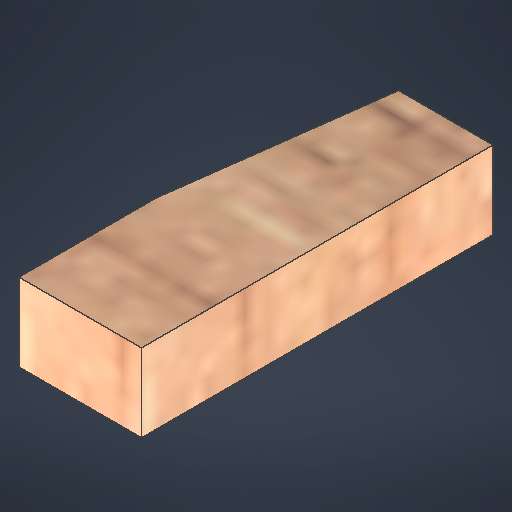
# Autodesk Inventor part: Stop Skiba
Saved by Autodesk Inventor 2027.1 (Build 311270010, 270A)
## iProperties
Created: 2025-11-09
Part Number: Stop Skiba
Material: Generic
Document SubType Name: Modeling
Designer: Nick
Density: 1 g/cm^3
Appearance: Birch - Natural Polished
Mass: 1.69348 g
Surface Area: 10.1101 cm^2
Volume: 1.69348 cm^3
Author: Nick
Autodesk Inventor part; units mm, degrees
ref_plane "YZ Plane" through (0, 0, 0) normal (1, 0, 0) x (0, 1, 0)
ref_plane "XZ Plane" through (0, 0, 0) normal (0, 1, 0) x (-1, 0, 0)
ref_plane "XY Plane" through (0, 0, 0) normal (0, 0, 1) x (1, 0, 0)
sketch "Sketch4" plane through (0, 0, 0) normal (0, 1, 0) x (-1, 0, 0)
  line L0 (5.0499, 10.8071) -> (-4.9501, 10.8071)
  line L1 (-4.9501, 10.8071) -> (-4.9501, -14.1929)
  line L2 (-4.9501, -14.1929) -> (5.0499, -14.1929)
  line L3 (5.0499, -14.1929) -> (5.0499, 10.8071)
  line L4 (5.0499, 3.3071) -> (-4.9501, 3.3071)
  line L5 (-4.9501, 3.3071) -> (-4.9501, 14.4921)
  line L6 (-4.9501, 14.4921) -> (5.0499, 14.4921)
  line L7 (5.0499, 14.4921) -> (5.0499, 3.3071)
  line L8 (5.0499, 3.3071) -> (2.7459, -14.1929)
  point P0 (0, 0)
  dimension "d12" = 10
  dimension "d13" = 25
  dimension "d14" = 10
  constraints: 18 end point, 4 parallel, 2 horizontal, 2 perpendicular, 1 point on line
  measures "d12" distance of L2.end L1.end
  measures "d13" distance of L1.end L0.end
  measures "d14" distance of L6.start L7.start
extrude "Extrusion7" add sketch "Sketch4" along normal blind 6.35 contours L3 L4 L1 L0 | L0 L5 L6 L7 | L8 L2 L1 L4
body "Solid4"
